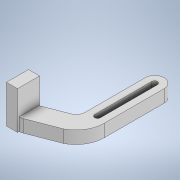
# Autodesk Inventor part: servo arm
Saved by Autodesk Inventor 2020 (Build 240168000, 168)
## iProperties
Created: 2022-02-17
Part Number: servo arm
Material: Generic
Document SubType Name: Modeling
Designer: rwte
Density: 1 g/cm^3
Appearance: Default
Author: rwte
## iProperties of the stored document _3DPrint.ipt
Created: 2022-02-19
Part Number: _3DPrint
Material: Generic
Document SubType Name: Modeling
Designer: rwte
Density: 1 g/cm^3
Appearance: Default
Author: rwte
Autodesk Inventor part; units mm, degrees
ref_plane "YZ Plane" through (0, 0, 0) normal (1, 0, 0) x (0, 1, 0)
ref_plane "XZ Plane" through (0, 0, 0) normal (0, 1, 0) x (-1, 0, 0)
ref_plane "XY Plane" through (0, 0, 0) normal (0, 0, 1) x (1, 0, 0)
sketch "Sketch1" plane through (0, 0, 0) normal (0, 1, 0) x (-1, 0, 0)
  line L0 (0, 0) -> (0, 19) construction
  line L1 (-3, 0) -> (-3, 19)
  line L2 (3, 19) -> (3, 0)
  arc A0 (-3, 0) -> (3, 0) centre (0, 0) ccw
  arc A1 (3, 19) -> (-3, 19) centre (0, 19) ccw construction
  line L3 (0, 19) -> (3, 24.1962) construction
  line L4 (2.5981, 17.5) -> (5.5981, 22.6962) construction
  line L5 (0.4019, 25.6962) -> (-2.5981, 20.5) construction
  arc A2 (-2.5981, 20.5) -> (2.5981, 17.5) centre (0, 19) ccw construction
  arc A3 (5.5981, 22.6962) -> (0.4019, 25.6962) centre (3, 24.1962) ccw construction
  line L6 (3, 24.1962) -> (12.2269, 27.738) construction
  line L7 (2.8111, 20.9102) -> (13.302, 24.9373) construction
  line L8 (11.1518, 30.5388) -> (1.9249, 26.9969) construction
  arc A4 (1.9249, 26.9969) -> (1.5, 21.5981) centre (3, 24.1962) ccw construction
  arc A5 (13.302, 24.9373) -> (11.1518, 30.5388) centre (12.2269, 27.738) ccw
  line L9 (12.2269, 27.738) -> (21.2256, 27.8951) construction
  arc A6 (5.0669, 21.7761) -> (3, 19) centre (5.8978, 19) ccw
  line L10 (5.0669, 21.7761) -> (13.302, 24.9373)
  line L11 (1.9249, 26.9969) -> (11.1518, 30.5388)
  arc A7 (1.9249, 26.9969) -> (-3, 19) centre (5.955, 19) ccw
  point P0 (0, 9.5)
  point P1 (1.5, 21.5981)
  point P2 (-2.5981, 20.5)
  point P3 (3, 18.1962)
  point P4 (7.6135, 25.9671)
  point P5 (1.9249, 26.9969)
  point P6 (16.7262, 27.8166)
  dimension "d0" = 6
  dimension "d5" = 25
  dimension "d6" = 150
  dimension "d7" = 6
  dimension "d8" = 12
  dimension "d9" = 12
  dimension "d10" = 111
  dimension "d11" = 200
  dimension "d13" = 9
  constraints: 32 end point, 18 point on circle, 14 tangent, 8 centre point, 5 midpoint, 3 parallel, 2 collinear, 2 point on line, 1 coincident, 1 concentric, 1 vertical
  measures "d0" distance of L1.start L2.end
  measures "d6" angle of L0 L3
  measures "d7" distance between parallel lines of L5 L4
  measures "d9" distance of L5.start L6.end
  measures "d10" angle of L0 L6
  measures "d13" distance of L6.end L9.end
extrude "Extrusion1" add sketch "Sketch1" along normal mid plane 4
sketch "Sketch2" plane through (0, 2, 0) normal (0, 1, 0) x (1, 0, 0)
  line L0 (0, 0) -> (0, -18.1) construction
  line L1 (-0.9, 0) -> (-0.9, -18.1)
  line L2 (0.9, -18.1) -> (0.9, 0)
  arc A0 (0.9, 0) -> (-0.9, 0) centre (0, 0) ccw
  arc A1 (-0.9, -18.1) -> (0.9, -18.1) centre (0, -18.1) ccw
  point P0 (0, -9.05)
  point P1 (-3, -19)
  point P2 (0, -19)
  dimension "d14" = 1.8
  constraints: 8 end point, 5 point on circle, 4 tangent, 2 centre point, 1 horizontal alignment, 1 midpoint, 1 parallel, 1 vertical
  measures "d14" distance of L2.end L1.start
extrude "Extrusion2" cut sketch "Sketch2" against normal through all
sketch "Sketch3" plane through (0, 0, 0) normal (0, 1, 0) x (-1, 0, 0)
  line L0 (-0.9, 0) -> (-0.9, 18.1) projected
  arc A0 (0.9, 18.1) -> (-0.9, 18.1) centre (0, 18.1) ccw projected
  line L1 (0.9, 18.1) -> (0.9, 0) projected
  arc A1 (-0.9, 0) -> (0.9, 0) centre (0, 0) ccw projected
  arc A2 (-3, 0) -> (3, 0) centre (0, 0) ccw projected
  line L2 (3, 0) -> (3, 19) projected
  arc A3 (5.0669, 21.7761) -> (3, 19) centre (5.8978, 19) ccw projected
  line L3 (5.0669, 21.7761) -> (13.302, 24.9373) projected
  arc A4 (13.302, 24.9373) -> (11.1518, 30.5388) centre (12.2269, 27.738) ccw projected
  line L4 (11.1518, 30.5388) -> (1.9249, 26.9969) projected
  arc A5 (1.9249, 26.9969) -> (-3, 19) centre (5.955, 19) ccw projected
  line L5 (-3, 19) -> (-3, 0) projected
  line L6 (15.7269, 24.238) -> (12.2269, 24.238)
  line L7 (12.2269, 24.238) -> (12.2269, 31.238)
  line L8 (12.2269, 31.238) -> (15.7269, 31.238)
  line L9 (15.7269, 31.238) -> (15.7269, 24.238)
  line L10 (13.9769, 24.238) -> (13.9769, 31.238) construction
  line L11 (12.2269, 27.738) -> (15.7269, 27.738) construction
  dimension "d17" = 7
  dimension "d18" = 3.5
  constraints: 12 end point, 4 midpoint, 2 parallel, 1 coincident, 1 horizontal, 1 perpendicular
  measures "d17" distance of L6.end L7.end
  measures "d18" distance of L6.start L6.end
extrude "Extrusion3" add sketch "Sketch3" along normal blind 10 and the other way blind 2 contours L7 A4 L3 | L3 A4 L7 L8 L9 L6
sketch "Sketch5" plane through (0, 2, 0) normal (0, 1, 0) x (1, 0, 0)
  point P0 (0, 0)
equation "\"d7\" = d0"
body "Solid1"
